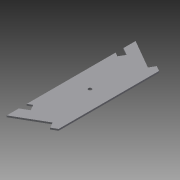
# Autodesk Inventor part: Triangle End
Saved by Autodesk Inventor 2015 SP1 (Build 190203100, 203)
## iProperties
Created: 2016-03-22
Part Number: Triangle End
Material: Generic
Document SubType Name: Modeling
Designer: Mac
Density: 1 g/cm^3
Appearance: Default
Author: Mac
Autodesk Inventor part; units mm, degrees
ref_plane "YZ Plane" through (0, 0, 0) normal (1, 0, 0) x (0, 1, 0)
ref_plane "XZ Plane" through (0, 0, 0) normal (0, 1, 0) x (-1, 0, 0)
ref_plane "XY Plane" through (0, 0, 0) normal (0, 0, 1) x (1, 0, 0)
sketch "Sketch1" plane through (0, 0, 0) normal (0, 1, 0) x (-1, 0, 0)
  line L0 (4.1559, 203.2) -> (4.1559, -203.2)
  line L1 (4.1559, -203.2) -> (156.5559, -291.1882)
  line L2 (4.1559, 203.2) -> (156.5559, 291.1882)
  line L3 (4.1559, 203.2) -> (180.1322, 203.2) construction
  line L4 (156.5559, 291.1882) -> (156.5559, -291.1882)
  point P0 (0, 0)
  point P1 (4.1559, 0)
  dimension "d0" = 120
  dimension "d1" = 30
  dimension "d2" = 406.4
  dimension "d5" = 152.4
  constraints: 10 end point, 2 vertical, 1 equal length, 1 horizontal, 1 horizontal alignment, 1 midpoint
  measures "d0" angle of L1 L0
  measures "d1" angle of L3 L2
  measures "d2" distance of L0.start L0.end
  measures "d5" distance between parallel lines of L0 L4
extrude "Extrusion1" add sketch "Sketch1" along normal blind 6.35
sketch "Sketch4" plane through (0, 6.35, 0) normal (0, 1, 0) x (1, 0, 0)
  line L0 (-4.1559, -203.2) -> (-4.1559, 203.2) projected
  point P0 (0, 0)
  point P1 (-80.3559, 0)
  dimension "d12" = 76.2
  dimension "d13" = 203.2
  measures "d12" distance from line of L0 point (-80.356, 0)
  measures "d13" vertical distance of L0.end point (-80.356, 0)
hole "Hole1" at (-80.3559, 6.35, 0) direction (0, -1, 0) diameter 13.4925 end through all
sketch "Sketch5" plane through (0, 6.35, 0) normal (0, 1, 0) x (1, 0, 0)
  line L0 (-1271.2154, -905.4078) -> (-39.3808, -194.2078) projected
  line L1 (-1258.5154, -927.4048) -> (-1271.2154, -905.4078) projected
  line L2 (-1258.5154, -927.4048) -> (-26.6808, -216.2048) projected
  line L3 (-39.3808, -194.2078) -> (-26.6808, -216.2048) projected
  circle A0 centre (-1049.6741, -711.3284) radius 3.3782 projected
  circle A1 centre (-248.9471, -249.0284) radius 3.3782 projected
  circle A2 centre (-318.2291, -289.0284) radius 3.3782 projected
  circle A3 centre (-1118.9562, -751.3284) radius 3.3782 projected
  line L4 (-127.679, -193.6709) -> (-1227.5312, -828.6709) projected
  line L5 (-140.379, -171.6739) -> (-127.679, -193.6709) projected
  line L6 (-140.379, -171.6739) -> (-1240.2312, -806.6739) projected
  line L7 (-1227.5312, -828.6709) -> (-1240.2312, -806.6739) projected
  circle A4 centre (-318.2291, 289.0284) radius 3.3782 projected
  circle A5 centre (-1118.9562, 751.3284) radius 3.3782 projected
  circle A6 centre (-1049.6741, 711.3284) radius 3.3782 projected
  circle A7 centre (-248.9471, 249.0284) radius 3.3782 projected
  line L8 (-1227.5312, 828.6709) -> (-127.679, 193.6709) projected
  line L9 (-1240.2312, 806.6739) -> (-1227.5312, 828.6709) projected
  line L10 (-1240.2312, 806.6739) -> (-140.379, 171.6739) projected
  line L11 (-127.679, 193.6709) -> (-140.379, 171.6739) projected
  line L12 (-39.3808, 194.2078) -> (-1271.2154, 905.4078) projected
  line L13 (-26.6808, 216.2048) -> (-39.3808, 194.2078) projected
  line L14 (-26.6808, 216.2048) -> (-1258.5154, 927.4048) projected
  line L15 (-1271.2154, 905.4078) -> (-1258.5154, 927.4048) projected
  line L16 (-156.5559, -291.1882) -> (-26.6808, -216.2048)
  line L17 (-39.3808, -194.2078) -> (-156.5559, -261.8588)
  line L18 (-156.5559, 291.1882) -> (-156.5559, -291.1882) projected
  line L19 (-156.5559, -261.8588) -> (-156.5559, -291.1882)
  line L20 (-156.5559, -210.343) -> (-127.679, -193.6709)
  line L21 (-127.679, -193.6709) -> (-140.379, -171.6739)
  line L22 (-140.379, -171.6739) -> (-156.5559, -181.0136)
  line L23 (-156.5559, -181.0136) -> (-156.5559, -210.343)
  line L24 (-39.3808, -194.2078) -> (-26.6808, -216.2048)
  line L25 (-156.5559, 181.0136) -> (-140.379, 171.6739)
  line L26 (-140.379, 171.6739) -> (-127.679, 193.6709)
  line L27 (-127.679, 193.6709) -> (-156.5559, 210.343)
  line L28 (-156.5559, 210.343) -> (-156.5559, 181.0136)
  line L29 (-156.5559, 261.8588) -> (-39.3808, 194.2078)
  line L30 (-39.3808, 194.2078) -> (-26.6808, 216.2048)
  line L31 (-4.1559, 203.2) -> (-156.5559, 291.1882) projected
  line L32 (-26.6808, 216.2048) -> (-156.5559, 291.1882)
  line L33 (-156.5559, 291.1882) -> (-156.5559, 261.8588)
  line L34 (-156.5559, 291.1882) -> (-26.6808, 216.2048)
  line L35 (-25.293, -216.5767) -> (-157.5719, -292.9479)
  line L36 (-157.5719, -292.9479) -> (-157.5719, -261.2722)
  line L37 (-157.5719, -261.2722) -> (-39.009, -192.8199)
  line L38 (-39.009, -192.8199) -> (-25.293, -216.5767)
  line L39 (-126.2911, -194.0428) -> (-157.5719, -212.1027)
  line L40 (-157.5719, -212.1027) -> (-157.5719, -180.427)
  line L41 (-157.5719, -180.427) -> (-140.0071, -170.286)
  line L42 (-140.0071, -170.286) -> (-126.2911, -194.0428)
  line L43 (-140.0071, 170.286) -> (-157.5719, 180.427)
  line L44 (-157.5719, 180.427) -> (-157.5719, 212.1027)
  line L45 (-157.5719, 212.1027) -> (-126.2911, 194.0428)
  line L46 (-126.2911, 194.0428) -> (-140.0071, 170.286)
  line L47 (-25.801, 215.6968) -> (-39.009, 192.8199)
  line L48 (-39.009, 192.8199) -> (-157.5719, 261.2722)
  line L49 (-157.5719, 261.2722) -> (-157.5719, 291.1882)
  line L50 (-25.801, 215.6968) -> (-156.5559, 291.1882)
  line L51 (-157.5719, 291.1882) -> (-157.5719, 291.7748)
  line L52 (-157.5719, 291.7748) -> (-156.5559, 291.1882)
  point P0 (0, 0)
  dimension "d22" = 1.016
  dimension "d23" = 1.016
  dimension "d24" = 1.016
  dimension "d25" = 1.016
  constraints: 70 end point, 14 collinear, 13 point on line, 2 perpendicular, 1 vertical, 11 other
  measures "d22" distance between parallel lines of L17 L37
  measures "d23" distance between parallel lines of L22 L41
  measures "d24" distance between parallel lines of L48 L29
  measures "d25" distance between parallel lines of L45 L27
extrude "Extrusion3" cut sketch "Sketch5" against normal blind 25.4 contours L18 L37 L38 L35 L36 L2 L3 L0 | L18 L2 L36 L0 | L0 L3 L2 L18 | L0 L36 L37 L18 | L36 L2 L1 L0 | L48 L49 L12 L18 | L18 L12 L13 L31 L47 L48 | L43 L44 L10 L18 | L18 L10 L11 L8 L45 L46 L43 | L39 L40 L4 L18 | L18 L4 L5 L6 L41 L42 L39 | L18 L6 L5 L4 | L4 L40 L6 L18 | L4 L7 L6 L40 | L6 L40 L41 L18 | L18 L8 L11 L10 | L10 L44 L8 L18 | L10 L9 L8 L44 | L8 L44 L45 L18 | L18 L14 L13 L12 | L12 L49 L51 L14 L18 | A0 | A1 | A2 | A3 | A4 | A5 | A6 | A7
body "Solid1"
